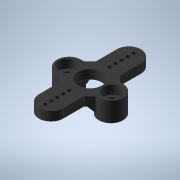
# Autodesk Inventor part: JointPlate5
Saved by Autodesk Inventor 2020 (Build 240168000, 168)
## iProperties
Created: 2019-04-02
Part Number: JointPlate5
Material: Generic
Document SubType Name: Modeling
Designer: mfans
Density: 1 g/cm^3
Appearance: Default
Author: mfans
Autodesk Inventor part; units mm, degrees
ref_plane "YZ Plane" through (0, 0, 0) normal (1, 0, 0) x (0, 1, 0)
ref_plane "XZ Plane" through (0, 0, 0) normal (0, 1, 0) x (-1, 0, 0)
ref_plane "XY Plane" through (0, 0, 0) normal (0, 0, 1) x (1, 0, 0)
sketch "Sketch1" plane through (0, 0, 0) normal (0, 1, 0) x (-1, 0, 0)
  line L0 (4, -17) -> (-4, -17)
  line L1 (-4, -17) -> (-4, 0)
  line L2 (-4, 0) -> (4, 0)
  line L3 (4, 0) -> (4, -17)
  line L4 (4, -17) -> (-4, 0) construction
  line L5 (-4, -17) -> (4, 0) construction
  point P0 (0, 0)
  point P1 (0, -8.5)
  dimension "d0" = 8
  dimension "d1" = 17
  dimension "d19" = 0
  dimension "d20" = 0
  constraints: 12 end point, 2 midpoint, 2 parallel, 1 horizontal, 1 perpendicular
  measures "d0" distance of L1.end L2.end
  measures "d1" distance of L0.end L1.end
  measures "d19" horizontal distance of point (0, 0) point (0, -8.5)
  measures "d20" distance from line of point (0, 0) L2
extrude "Extrusion1" add sketch "Sketch1" along normal mid plane 4
sketch "Sketch2" plane through (0, 2, 0) normal (0, 1, 0) x (1, 0, 0)
  line L0 (-4, 17) -> (-4, 0) projected
  line L1 (-4, 0) -> (4, 0) projected
  line L2 (4, 0) -> (4, 17) projected
  line L3 (4, 17) -> (-4, 17) projected
  point P0 (0, 0)
  point P1 (0, 6.75)
  point P2 (0, 8.75)
  point P3 (0, 10.75)
  point P4 (0, 12.75)
  point P5 (0, 14.75)
  dimension "d4" = 6.75
  dimension "d7" = 2
  constraints: 1 vertical, 4 other
  measures "d4" distance of point (0, 0) point (0, 6.75)
  measures "d7" distance of point (0, 6.75) point (0, 8.75)
hole "Hole1" at (0, 2, -6.75) at (0, 2, -8.75) at (0, 2, -10.75) at (0, 2, -12.75) at (0, 2, -14.75) direction (0, -1, 0) diameter 1.5 end through all
fillet "Fillet1" radius 4 2 edges at (-4, 0, -17) (4, 0, -17)
mirror "Mirror1" about plane through (0, 0, 0) normal (0, 0, 1) of "Extrusion1", "Hole1", "Fillet1"
sketch "Sketch3" plane through (0, 2, 0) normal (0, 1, 0) x (1, 0, 0)
  line L0 (11, -4) -> (4, -4)
  line L1 (4, -4) -> (4, 4)
  line L2 (4, 4) -> (11, 4)
  line L3 (11, 4) -> (11, -4)
  line L4 (11, -4) -> (4, 4) construction
  line L5 (4, -4) -> (11, 4) construction
  line L6 (4, 13) -> (4, -13) projected
  point P0 (0, 0)
  point P1 (7.5, 0)
  point P2 (4, -14)
  dimension "d22" = 0
  dimension "d23" = 0
  dimension "d24" = 8
  dimension "d25" = 7.5
  constraints: 12 end point, 2 midpoint, 2 parallel, 1 horizontal, 1 perpendicular
  measures "d22" vertical distance of point (0, 0) point (7.5, 0)
  measures "d23" distance between parallel lines of L6 L1
  measures "d24" distance of L2.end L0.start
  measures "d25" distance of point (0, 0) point (7.5, 0)
extrude "Extrusion2" add sketch "Sketch3" against normal blind 4
fillet "Fillet2" radius 4 2 edges at (11, 0, -4) (11, 0, 4)
sketch "Sketch4" plane through (0, 2, 0) normal (0, 1, 0) x (1, 0, 0)
  point P0 (0, 0)
  point P1 (7.5, 0)
  dimension "d29" = 7.5
  measures "d29" distance of point (0, 0) point (7.5, 0)
hole "Hole2" at (7.5, 2, 0) direction (0, -1, 0) diameter 4 end through all
mirror "Mirror2" about plane through (0, 0, 0) normal (1, 0, 0) of "Extrusion2", "Fillet2", "Hole2"
sketch "Sketch5" plane through (0, 2, 0) normal (0, 1, 0) x (1, 0, 0)
  circle A0 centre (0, 0) radius 4
  dimension "d37" = 8
  constraints: 1 centre point, 1 coincident
  measures "d37" diameter of A0
extrude "Extrusion3" cut sketch "Sketch5" against normal through all
chamfer "Chamfer1" distance 2 angle 45 4 edges at (4, 0, 4) (-4, 0, 4) (-4, 0, -4) (4, 0, -4)
sketch "Sketch6" plane through (0, 2, 0) normal (0, 1, 0) x (1, 0, 0)
  circle A0 centre (0, 0) radius 4 projected
  circle A1 centre (-7.5, 0) radius 2 projected
  arc A2 (-7, 4) -> (-7, -4) centre (-7, 0) ccw projected
  line L0 (-6, -4) -> (-7, -4) projected
  line L1 (-4, -6) -> (-6, -4) projected
  line L2 (-4, -6) -> (-4, -13) projected
  arc A3 (-4, -13) -> (4, -13) centre (0, -13) ccw projected
  line L3 (4, -6) -> (4, -13) projected
  line L4 (6, -4) -> (4, -6) projected
  line L5 (6, -4) -> (7, -4) projected
  arc A4 (7, -4) -> (7, 4) centre (7, 0) ccw projected
  line L6 (7, 4) -> (6, 4) projected
  line L7 (4, 6) -> (6, 4) projected
  line L8 (4, 13) -> (4, 6) projected
  arc A5 (4, 13) -> (-4, 13) centre (0, 13) ccw projected
  line L9 (-4, 13) -> (-4, 6) projected
  line L10 (-6, 4) -> (-4, 6) projected
  line L11 (-7, 4) -> (-6, 4) projected
  circle A6 centre (7.5, 0) radius 2 projected
  circle A7 centre (0, 12.75) radius 0.75 projected
  circle A8 centre (0, 8.75) radius 0.75 projected
  circle A9 centre (0, 6.75) radius 0.75 projected
  circle A10 centre (0, 10.75) radius 0.75 projected
  circle A11 centre (0, 14.75) radius 0.75 projected
  circle A12 centre (0, -8.75) radius 0.75 projected
  circle A13 centre (0, -6.75) radius 0.75 projected
  circle A14 centre (0, -10.75) radius 0.75 projected
  circle A15 centre (0, -14.75) radius 0.75 projected
  circle A16 centre (0, -12.75) radius 0.75 projected
  circle A17 centre (-7.5, 0) radius 3
  circle A18 centre (7.5, 0) radius 3
  dimension "d43" = 6
  dimension "d44" = 6
  constraints: 2 centre point, 2 coincident
  measures "d43" diameter of A17
  measures "d44" diameter of A18
extrude "Extrusion4" cut sketch "Sketch6" against normal blind 2.5 contours A17 | A18
sketch "Sketch7" plane through (0, -2, 0) normal (0, -1, 0) x (1, 0, 0)
  circle A0 centre (7.5, 0) radius 2 projected
  arc A1 (7, -4) -> (7, 4) centre (7, 0) ccw projected
  circle A2 centre (-7.5, 0) radius 2 projected
  circle A3 centre (0, 0) radius 4 projected
  circle A4 centre (-7.5, 0) radius 2 projected
  circle A5 centre (7.5, 0) radius 2 projected
  arc A6 (-7, 4) -> (-7, -4) centre (-7, 0) ccw projected
  line L0 (-6, -4) -> (-7, -4) projected
  line L1 (-4, -6) -> (-6, -4) projected
  line L2 (-4, -13) -> (-4, -6) projected
  arc A7 (-4, -13) -> (4, -13) centre (0, -13) ccw projected
  line L3 (4, -13) -> (4, -6) projected
  line L4 (6, -4) -> (4, -6) projected
  line L5 (6, -4) -> (7, -4) projected
  arc A8 (7, -4) -> (7, 4) centre (7, 0) ccw projected
  line L6 (7, 4) -> (6, 4) projected
  line L7 (4, 6) -> (6, 4) projected
  line L8 (4, 6) -> (4, 13) projected
  arc A9 (4, 13) -> (-4, 13) centre (0, 13) ccw projected
  line L9 (-4, 6) -> (-4, 13) projected
  line L10 (-6, 4) -> (-4, 6) projected
  line L11 (-7, 4) -> (-6, 4) projected
  circle A10 centre (0, -12.75) radius 0.75 projected
  circle A11 centre (0, -8.75) radius 0.75 projected
  circle A12 centre (0, -6.75) radius 0.75 projected
  circle A13 centre (0, -10.75) radius 0.75 projected
  circle A14 centre (0, -14.75) radius 0.75 projected
  circle A15 centre (0, 8.75) radius 0.75 projected
  circle A16 centre (0, 6.75) radius 0.75 projected
  circle A17 centre (0, 10.75) radius 0.75 projected
  circle A18 centre (0, 14.75) radius 0.75 projected
  circle A19 centre (0, 12.75) radius 0.75 projected
  arc A20 (4, -2.6458) -> (4, 2.6458) centre (7, 0) ccw
  arc A21 (-4, 2.6458) -> (-4, -2.6458) centre (-7, 0) ccw
  line L12 (4, 2.6458) -> (4, -2.6458)
  circle A22 centre (0, 0) radius 4 projected
  line L13 (4, -13) -> (4, -6) projected
  line L14 (-4, 2.6458) -> (-4, -2.6458)
  point P0 (7, 4)
  constraints: 4 end point, 4 point on circle, 3 vertical, 2 centre point, 2 coincident, 1 collinear, 1 concentric, 1 tangent, 1 other
extrude "Extrusion5" add sketch "Sketch7" along normal blind 2 contours A20 L12 A1 | L14 A21 A6
thicken "Thicken1" operation add thickness 1 both sides no extend neighbours yes toward (0, -1, 0) faces at (2.9148, 2, 9.2802)
thicken "Thicken2" operation add thickness 1.5 both sides no extend neighbours yes toward (0, -1, 0) faces at (10.1327, -0.5, 0.3197)
thicken "Thicken3" operation add thickness 1.5 both sides no extend neighbours yes toward (0, -1, 0) faces at (-4.8673, -0.5, 0.3197)
sketch "Sketch8" plane through (0, -4, 0) normal (0, -1, 0) x (1, 0, 0)
  arc A0 (-4, 2.6458) -> (-4, -2.6458) centre (-7, 0) ccw projected
  line L0 (-4, -2.6458) -> (-4, 2.6458) projected
  circle A1 centre (-7.5, 0) radius 2 projected
  arc A2 (4, -2.6458) -> (4, 2.6458) centre (7, 0) ccw projected
  line L1 (4, 2.6458) -> (4, -2.6458) projected
  circle A3 centre (7.5, 0) radius 2 projected
  point P0 (0, 0)
extrude "Extrusion6" add sketch "Sketch8" along normal blind 1.5
chamfer "Chamfer2" distance 2 angle 45 4 edges at (5.3543, -2, 3.6458) (5.3543, -2, -3.6458) (-5.3543, -2, -3.6458) (-5.3543, -2, 3.6458)
body "Solid1"
